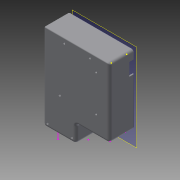
# Autodesk Inventor part: arduino-holder
Saved by Autodesk Inventor 2014 (Build 180170000, 170)
## iProperties
Created: 2017-08-03
Part Number: arduino-holder
Material: 一般
Document SubType Name: Modeling
Designer: hide
Density: 1 g/cm^3
Appearance: 既定
Author: hide
Autodesk Inventor part; units mm, degrees
ref_plane "YZ Plane" through (0, 0, 0) normal (1, 0, 0) x (0, 1, 0)
ref_plane "XY Plane" through (0, 0, 0) normal (0, 0, 1) x (1, 0, 0)
sketch "スケッチ1" plane through (0, 0, 0) normal (0, 1, 0) x (-1, 0, 0)
  line L0 (0, 0) -> (73, 0)
  line L1 (73, 0) -> (73, -76.4)
  line L2 (0, -76) -> (0, 0)
  circle A0 centre (21.8, -5) radius 1.3
  circle A1 centre (50, -5) radius 1.3
  circle A2 centre (55, -57) radius 1.3
  circle A3 centre (15, -15) radius 1.3
  circle A4 centre (15, -55) radius 1.3
  line L3 (4.5, -3) -> (58, -3)
  line L4 (58, -3) -> (58, -73)
  line L5 (58, -73) -> (4.5, -73)
  line L6 (4.5, -73) -> (4.5, -3)
  line L7 (73, -12.2504) -> (60, -12.2504)
  line L8 (60, -12.2504) -> (60, -2.9504)
  line L9 (60, -2.9504) -> (73, -2.9504)
  line L10 (73, -2.9504) -> (73, -12.2504)
  line L11 (37, -76) -> (37, -95.2)
  line L12 (37, -95.2) -> (73, -95.2)
  line L13 (73, -95.2) -> (73, -76.4)
  line L14 (39, -73.2) -> (71, -73.2)
  line L15 (71, -73.2) -> (71, -93.2)
  line L16 (71, -93.2) -> (39, -93.2)
  line L17 (39, -93.2) -> (39, -73.2)
  circle A5 centre (41.6, -75.8) radius 1.3
  circle A6 centre (41.6, -90.6) radius 1.3
  circle A7 centre (68.4, -75.8) radius 1.3
  circle A8 centre (68.4, -90.6) radius 1.3
  line L18 (0, -76) -> (37, -76)
  dimension "d0" = 0
  dimension "d1" = 28.2
  dimension "d2" = 5
  dimension "d3" = 2.6
  dimension "d4" = 2.6
  dimension "d5" = 2.6
  dimension "d13" = 52
  dimension "d14" = 0
  dimension "d15" = 40
  dimension "d16" = 2.6
  dimension "d17" = 2.6
  dimension "d20" = 70
  dimension "d21" = 2
  dimension "d22" = 53.5
  dimension "d23" = 3
  dimension "d24" = 9.3
  dimension "d31" = 15
  dimension "d32" = 15
  dimension "d92" = 4.5
  dimension "d93" = 3
  dimension "d94" = 15
  dimension "d110" = 76.4
  dimension "d111" = 32
  dimension "d114" = 2
  dimension "d115" = 2
  dimension "d118" = 2.6
  dimension "d121" = 2.6
  dimension "d122" = 2.6
  dimension "d123" = 2.6
  dimension "d124" = 2.6
  dimension "d125" = 2.6
  dimension "d126" = 2.6
  dimension "d127" = 2.6
  dimension "d128" = 2.6
  dimension "d129" = 2.6
  dimension "d134" = 13
  dimension "d135" = 2
  dimension "d147" = 3
  dimension "d148" = 0.2
  dimension "d149" = 20
  dimension "d150" = 2.6
  dimension "d151" = 2.6
  constraints: 38 end point, 9 centre point, 8 parallel, 5 perpendicular, 4 horizontal, 1 point on line
  measures "d0" vertical distance of A1.centre A0.centre
  measures "d1" distance of A0.centre A1.centre
  measures "d2" horizontal distance of A2.centre A1.centre
  measures "d3" diameter of A0
  measures "d4" diameter of A1
  measures "d5" diameter of A2
  measures "d13" vertical distance of A2.centre A1.centre
  measures "d14" horizontal distance of A4.centre A3.centre
  measures "d15" distance of A3.centre A4.centre
  measures "d16" diameter of A3
  measures "d17" diameter of A4
  measures "d20" distance of L3.end L4.end
  measures "d21" distance from line of L3 A1.centre
  measures "d22" distance between parallel lines of L4 L6
  measures "d23" distance from line of L4 A2.centre
  measures "d24" distance between parallel lines of L7 L9
  measures "d31" distance from line of L0 A3.centre
  measures "d32" distance from line of L2 A3.centre
  measures "d92" distance between parallel lines of L2 L6
  measures "d93" distance between parallel lines of L0 L3
  measures "d94" distance between parallel lines of L1 L4
  measures "d110" distance of L0.end L1.end
  measures "d111" distance between parallel lines of L15 L17
  measures "d114" distance between parallel lines of L16 L12
  measures "d115" distance between parallel lines of L17 L11
  measures "d118" distance from line of L17 A5.centre
  measures "d121" distance from line of L15 A7.centre
  measures "d122" distance from line of L15 A8.centre
  measures "d123" distance from line of L16 A8.centre
  measures "d124" distance from line of L16 A6.centre
  measures "d125" distance from line of L17 A6.centre
  measures "d126" diameter of A7
  measures "d127" diameter of A5
  measures "d128" diameter of A6
  measures "d129" diameter of A8
  measures "d134" distance between parallel lines of L10 L8
  measures "d135" distance between parallel lines of L13 L15
  measures "d147" distance between parallel lines of L5 L18
  measures "d148" distance between parallel lines of L5 L14
  measures "d149" distance of L14.end L15.end
  measures "d150" distance from line of L14 A5.centre
  measures "d151" distance from line of L14 A7.centre
extrude "押し出し1" add sketch "スケッチ1" along normal blind 2 contours L0 L1 L9 L8 L7 L13 L12 L11 L18 L2 | L1 L7 L8 L9 | L3 L4 L5 L6 | L14 L15 L16 L17 | A5 | A7
sketch "スケッチ2" plane through (0, 2, 0) normal (0, 1, 0) x (1, 0, 0)
  circle A0 centre (-55, 57) radius 1.3 projected
  circle A1 centre (-50, 5) radius 1.3 projected
  circle A2 centre (-21.8, 5) radius 1.3 projected
  circle A3 centre (-55, 57) radius 2.7
  circle A4 centre (-50, 5) radius 2.7
  circle A5 centre (-21.8, 5) radius 2.7
  circle A6 centre (-15, 55) radius 1.3 projected
  circle A7 centre (-15, 15) radius 1.3 projected
  circle A8 centre (-15, 55) radius 2.8
  circle A9 centre (-15, 15) radius 2.8
  circle A10 centre (-41.6, 79) radius 1.3 projected
  circle A11 centre (-41.6, 90.6) radius 1.3 projected
  circle A12 centre (-68.4, 79) radius 1.3 projected
  circle A13 centre (-68.4, 90.6) radius 1.3 projected
  circle A14 centre (-68.4, 90.6) radius 2.7
  circle A15 centre (-68.4, 79) radius 2.7
  circle A16 centre (-41.6, 79) radius 2.7
  circle A17 centre (-41.6, 90.6) radius 2.7
  dimension "d8" = 1.4
  dimension "d9" = 1.4
  dimension "d10" = 1.4
  dimension "d18" = 1.5
  dimension "d19" = 1.5
  dimension "d130" = 1.4
  dimension "d131" = 1.4
  dimension "d132" = 1.4
  dimension "d133" = 1.4
  constraints: 9 centre point, 9 coincident
  measures "d8" radial gap between concentric circles of A3 A0
  measures "d9" radial gap between concentric circles of A1 A4
  measures "d10" radial gap between concentric circles of A5 A2
  measures "d18" radial gap between concentric circles of A8 A6
  measures "d19" radial gap between concentric circles of A7 A9
  measures "d130" radial gap between concentric circles of A14 A13
  measures "d131" radial gap between concentric circles of A12 A15
  measures "d132" radial gap between concentric circles of A16 A10
  measures "d133" radial gap between concentric circles of A17 A11
extrude "押し出し2" add sketch "スケッチ2" along normal blind 7 contours A3 | A4 | A5 | A14 | A17
sketch "スケッチ3" plane through (0, 2, 0) normal (0, 1, 0) x (1, 0, 0)
  line L0 (-73, 0) -> (0, 0) projected
  line L1 (0, 0) -> (0, 76) projected
  line L2 (0, 75.4) -> (0, 0)
  line L3 (0, 0) -> (-60, 0)
  line L4 (-38.3, 75.1) -> (-1.3, 75.1)
  line L5 (-1.3, 75.1) -> (-1.3, 1.3)
  line L6 (-1.3, 1.3) -> (-70.631, 1.3)
  line L7 (-73, 95.2) -> (-70.631, 95.2)
  line L8 (-73, 78.8) -> (-73, 95.2)
  line L9 (-70.631, 95.2) -> (-37, 95.2)
  line L10 (-24, 75.1) -> (-38.3, 75.1)
  line L11 (-73, 95.2) -> (-73, 0) projected
  line L12 (-73, 95.2) -> (-71.7, 95.2)
  line L13 (-71.7, 95.2) -> (-71.7, 0)
  line L14 (-71.7, 0) -> (-73, 0)
  line L15 (-73, 0) -> (-73, 95.2)
  line L16 (-73, 0) -> (0, 0)
  line L17 (0, 0) -> (0, 1.3)
  line L18 (0, 1.3) -> (-73, 1.3)
  line L19 (-73, 1.3) -> (-73, 0)
  line L20 (0, 0) -> (-1.3, 0)
  line L21 (-1.3, 0) -> (-1.3, 76)
  line L22 (-1.3, 76) -> (0, 76)
  line L23 (0, 76) -> (0, 0)
  line L24 (-38.3, 76) -> (-38.3, 74.7)
  line L25 (-38.3, 74.7) -> (0, 74.7)
  line L26 (0, 74.7) -> (0, 76)
  line L27 (-37, 95.2) -> (-38.9, 95.2)
  line L28 (-38.3, 74.7) -> (-36.4, 74.7)
  line L29 (-37, 95.2) -> (-73, 95.2)
  line L30 (-73, 95.2) -> (-73, 93.9)
  line L31 (-73, 93.9) -> (-37, 93.9)
  line L32 (-37, 93.9) -> (-37, 95.2)
  circle A0 centre (-41.6, 90.6) radius 2.7 projected
  circle A1 centre (-21.8, 5) radius 2.7 projected
  circle A2 centre (-55, 57) radius 2.7 projected
  circle A3 centre (-50, 5) radius 2.7 projected
  circle A4 centre (-68.4, 90.6) radius 2.7 projected
  circle A5 centre (-15, 55) radius 1.3 projected
  line L33 (-73, 0) -> (0, 0) projected
  line L34 (0, 0) -> (0, 76) projected
  line L35 (-37, 76) -> (-37, 95.2) projected
  line L36 (-37, 95.2) -> (-73, 95.2) projected
  line L37 (-73, 95.2) -> (-73, 0) projected
  line L38 (-37, 95.2) -> (-38.3, 95.2)
  line L39 (-38.3, 95.2) -> (-38.3, 74.7)
  line L40 (-38.3, 74.7) -> (-37, 74.7)
  line L41 (-37, 74.7) -> (-37, 95.2)
  line L42 (0, 76) -> (-37, 76) projected
  line L43 (-38.3, 74.7) -> (0, 74.7)
  line L44 (0, 74.7) -> (0, 76)
  line L45 (0, 76) -> (-38.3, 76)
  line L46 (-38.3, 76) -> (-38.3, 74.7)
  dimension "d27" = 1.3
  dimension "d28" = 1.3
  dimension "d136" = 1.3
  dimension "d137" = 1.3
  dimension "d138" = 1.3
  dimension "d139" = 1.3
  dimension "d141" = 1.3
  dimension "d152" = 0
  dimension "d153" = 1.3
  constraints: 76 end point, 15 parallel, 10 horizontal, 7 perpendicular, 4 point on line
  measures "d27" distance between parallel lines of L1 L5
  measures "d28" distance between parallel lines of L6 L0
  measures "d136" distance between parallel lines of L29 L31
  measures "d137" distance between parallel lines of L11 L13
  measures "d138" distance between parallel lines of L18 L0
  measures "d139" distance between parallel lines of L2 L21
  measures "d141" distance between parallel lines of L41 L39
  measures "d152" distance between parallel lines of L22 L42
  measures "d153" distance between parallel lines of L45 L43
extrude "押し出し3" add sketch "スケッチ3" along normal blind 25 contours L11 L18 L13 L0 | L13 L18 L6 L21 L0 | L11 L8 L31 L13 L18 | L21 L18 L1 L0 | L31 L8 L7 L13 | L13 L7 L9 L39 L31 | L5 L25 L1 L18 | L39 L9 L32 L31 | L31 L35 L45 L39 | L25 L41 L4 L5 | L5 L21 L22 L1 L25 | L45 L41 L4 L24 | L4 L41 L42 L21 | L4 L41 L25 L24
sketch "スケッチ4" plane through (0, 2, 0) normal (0, 1, 0) x (1, 0, 0)
  line L0 (-1.3, 1.3) -> (-1.3, 75.1) projected
  line L1 (-1.3, 75.1) -> (-38.3, 75.1) projected
  line L2 (-58.7, 102.1) -> (-58.7, 1.3) projected
  line L3 (-58.7, 1.3) -> (-1.3, 1.3) projected
  circle A0 centre (-20, 15) radius 2.8 projected
  circle A1 centre (-21.8, 5) radius 2.7 projected
  circle A2 centre (-55, 57) radius 2.7 projected
  circle A3 centre (-50, 5) radius 2.7 projected
  circle A4 centre (-20, 55) radius 2.8 projected
  point P0 (-58.7, 85.7)
  point P1 (0, 0)
  point P2 (-25.3, 85.7)
  point P3 (-58.7, 87)
  constraints: 1 other
sketch "スケッチ5" plane through (0, 2, 0) normal (0, 1, 0) x (1, 0, 0)
  circle A0 centre (-15, 55) radius 1.3 projected
  circle A1 centre (-15, 15) radius 1.3 projected
  circle A2 centre (-15, 55) radius 3
  circle A3 centre (-15, 15) radius 3
  point P0 (0, 0)
  dimension "d33" = 6
  dimension "d34" = 6
  constraints: 2 centre point, 2 coincident
  measures "d33" diameter of A2
  measures "d34" diameter of A3
extrude "押し出し4" add sketch "スケッチ5" along normal blind 5
sketch "スケッチ7" plane through (0, 2, 0) normal (0, 1, 0) x (1, 0, 0)
  line L0 (-58.7, 1.3) -> (-1.3, 1.3) projected
  line L1 (-58.7, 1.3) -> (-48, 1.3)
  line L2 (-48, 1.3) -> (-48, 11.3)
  line L3 (-48, 11.3) -> (-58.7, 11.3)
  line L4 (-58.7, 11.3) -> (-58.7, 1.3)
  line L5 (-58.7, 1.3) -> (-46.5, 1.3)
  line L6 (-46.5, 1.3) -> (-46.5, 12.8)
  line L7 (-46.5, 12.8) -> (-58.7, 12.8)
  line L8 (-58.7, 12.8) -> (-58.7, 1.3)
  line L9 (-71.7, 1.3) -> (-61, 1.3)
  line L10 (-61, 1.3) -> (-61, 11.3)
  line L11 (-61, 11.3) -> (-71.7, 11.3)
  line L12 (-71.7, 11.3) -> (-71.7, 1.3)
  line L13 (-71.7, 1.3) -> (-59.5, 1.3)
  line L14 (-59.5, 1.3) -> (-59.5, 12.8)
  line L15 (-59.5, 12.8) -> (-71.7, 12.8)
  line L16 (-71.7, 12.8) -> (-71.7, 1.3)
  point P0 (0, 0)
  dimension "d43" = 10.7
  dimension "d44" = 10
  dimension "d45" = 1.5
  dimension "d46" = 1.5
  dimension "d143" = 10
  dimension "d144" = 1.5
  dimension "d145" = 10.7
  dimension "d146" = 1.5
  constraints: 32 end point, 8 parallel, 4 horizontal, 4 perpendicular
  measures "d43" distance between parallel lines of L2 L4
  measures "d44" distance between parallel lines of L0 L3
  measures "d45" distance between parallel lines of L7 L3
  measures "d46" distance between parallel lines of L6 L2
  measures "d143" distance between parallel lines of L11 L13
  measures "d144" distance between parallel lines of L15 L11
  measures "d145" distance between parallel lines of L16 L10
  measures "d146" distance between parallel lines of L10 L14
extrude "押し出し6" add sketch "スケッチ7" along normal blind 11 contours L10 L11 L16 L15 L14 L13
sketch "スケッチ8" plane through (0, 2, 0) normal (0, 1, 0) x (1, 0, 0)
  line L0 (-58.7, 11.3) -> (-65.1062, 11.3)
  line L1 (-65.1062, 11.3) -> (-65.1062, 1.3)
  line L2 (-65.1062, 1.3) -> (-58.7, 1.3)
  line L3 (-58.7, 1.3) -> (-48, 1.3) projected
  line L4 (-71.7, 11.3) -> (-77.9031, 11.3)
  line L5 (-77.9031, 11.3) -> (-77.9031, 1.3)
  line L6 (-77.9031, 1.3) -> (-71.7, 1.3)
  line L7 (-71.7, 1.3) -> (-71.7, 11.3)
  point P0 (0, 0)
  dimension "d54" = 0
  constraints: 14 end point, 3 parallel, 2 horizontal, 2 perpendicular
  measures "d54" distance between parallel lines of L2 L3
extrude "押し出し7" cut sketch "スケッチ8" against normal blind 11 and the other way blind 11.5
fillet "フィレット1" radius 5 2 edges at (-66.35, 2, -11.3) (-66.35, 2, -1.3)
ref_plane "作業平面1" through (0, 26.8, 0) normal (0, 1, 0) x (-1, 0, 0)
sketch "スケッチ9" plane through (0, 26.8, 0) normal (0, 1, 0) x (-1, 0, 0)
  circle A0 centre (3, -3) radius 0.75
  circle A1 centre (3, -3) radius 2.5
  circle A2 centre (70.0026, -50.581) radius 0.75
  circle A3 centre (70.0026, -50.581) radius 2.5
  line L0 (7.986, -75.1) -> (20.986, -75.1) projected
  line L1 (1.3, -1.3) -> (71.7, -1.3) projected
  line L2 (1.3, -75.1) -> (1.3, -1.3) projected
  circle A4 centre (3, -73.4) radius 0.75
  circle A5 centre (3, -73.4) radius 2.5
  circle A6 centre (70.0026, -3) radius 0.75
  circle A7 centre (70.0026, -3) radius 2.5
  line L3 (7.986, -75.1) -> (1.3, -75.1) projected
  line L4 (58.7, -102.1) -> (38.3, -102.1) projected
  line L5 (0, -76) -> (37, -76) projected
  line L6 (37, -76) -> (37, -95.2) projected
  line L7 (37, -95.2) -> (73, -95.2) projected
  line L8 (73, -95.2) -> (73, 0) projected
  line L9 (73, 0) -> (0, 0) projected
  line L10 (0, 0) -> (0, -76) projected
  line L11 (1.3, -74.7) -> (1.3, -1.3) projected
  line L12 (71.7, -1.3) -> (71.7, -93.9) projected
  line L13 (71.7, -93.9) -> (38.3, -93.9) projected
  line L14 (1.3, -1.3) -> (71.7, -1.3) projected
  line L15 (38.3, -93.9) -> (38.3, -74.7) projected
  line L16 (38.3, -74.7) -> (1.3, -74.7) projected
  point P0 (58.7, -85.7)
  point P1 (25.3, -85.7)
  point P2 (58.7, -87)
  dimension "d56" = 1.5
  dimension "d57" = 5
  dimension "d58" = 1.5
  dimension "d59" = 5
  dimension "d62" = 1.7
  dimension "d63" = 1.7
  dimension "d100" = 5
  dimension "d101" = 1.5
  dimension "d102" = 1.5
  dimension "d103" = 5
  dimension "d104" = 1.7
  dimension "d105" = 1.7
  dimension "d106" = 1.7
  constraints: 8 centre point, 4 coincident, 1 other
  measures "d56" diameter of A0
  measures "d57" diameter of A1
  measures "d58" diameter of A2
  measures "d59" diameter of A3
  measures "d62" distance from line of L1 A0.centre
  measures "d63" distance from line of L2 A0.centre
  measures "d100" diameter of A7
  measures "d101" diameter of A6
  measures "d102" diameter of A4
  measures "d103" diameter of A5
  measures "d104" distance from line of L2 A4.centre
  measures "d105" distance from line of A4.centre L3
  measures "d106" distance from line of L1 A6.centre
extrude "押し出し8" add sketch "スケッチ9" against normal blind 8 contours A1 L2 L1 | L1 L2 A1 | A7 L12 L1 | L1 L12 A7 | A5 L16 L2 | L2 L3 A5 | L16 A5 L3 L2 | L12 A3 | A3 L12
sketch "スケッチ11" plane through (0, 18.8, 0) normal (0, -1, 0) x (1, 0, 0)
  line L0 (-58.7, -3) -> (-58.7, -1.3) projected
  line L1 (-1.3, -75.1) -> (-5.5, -75.1) projected
  circle A0 centre (-70.0026, -50.581) radius 2.5 projected
  circle A1 centre (-70.0026, -50.581) radius 0.75 projected
  point P0 (-72.5026, -50.581)
  point P1 (-58.7, -85.7)
  point P2 (-72.5026, -50.581)
  point P3 (0, 0)
  point P4 (-5.5, -73.4)
  point P5 (-72.5026, -50.581)
  point P6 (-72.5026, -3)
  point P7 (-72.5026, -50.581)
  point P8 (-58.7, -1.3)
  constraints: 2 other
fillet "フィレット4" radius 3 12 edges at (0, 13.5, 0) (0, 0, -38) (-73, 0, -0.65) (-73, 0, -53.25) (-73, 13.5, 0) (-55, 0, -95.2) (-37, 0, -85.6) (-37, 13.5, -95.2) (-73, 13.5, -95.2) (-18.5, 0, -76) (0, 13.5, -76) (-37, 13.5, -76)
fillet "フィレット5" radius 1 3 edges at (-71.3964, 0.3448, -0.3448) (-0.8787, 0.8787, -0.8787) (-36.5, 0, 0)
sketch "スケッチ15" plane through (0, 3, -73.4) normal (1, 0, 0) x (0, 0, -1)
  line L0 (-73.4, 24) -> (-0.4, 24) projected
  line L1 (-73.4, 24) -> (-73.4, -2) projected
  line L2 (-64.5, 24) -> (-50.5, 24)
  line L3 (-50.5, 24) -> (-50.5, 18.8)
  line L4 (-50.5, 18.8) -> (-64.5, 18.8)
  line L5 (-64.5, 18.8) -> (-64.5, 24)
  point P0 (0, 24)
  point P1 (-73.4, -3)
  point P2 (2.6, 24)
  dimension "d95" = 14
  dimension "d96" = 5.2
  dimension "d97" = 8.9
  constraints: 8 end point, 2 parallel, 1 horizontal, 1 perpendicular, 1 point on line
  measures "d95" distance of L3.end L4.end
  measures "d96" distance of L4.end L2.start
  measures "d97" distance between parallel lines of L1 L5
extrude "押し出し12" cut sketch "スケッチ15" against normal blind 10
fillet "フィレット8" radius 1 6 edges at (-38.3, 14.5, -93.9) (-1.3, 10.4, -74.7) (-71.7, 14.5, -93.9) (-71.7, 16.15, -1.3) (-1.3, 10.4, -1.3) (-38.3, 14.5, -74.7)
sketch "スケッチ16" plane through (-3, 3, -76) normal (0, 0, -1) x (-1, 0, 0)
  line L0 (0, 24) -> (31, 24) projected
  line L1 (-3, 24) -> (-3, 0) projected
  line L2 (9, 24) -> (22, 24)
  line L3 (22, 24) -> (22, 7)
  line L4 (22, 7) -> (9, 7)
  line L5 (9, 7) -> (9, 24)
  point P0 (-3, -3)
  dimension "d155" = 12
  dimension "d156" = 13
  dimension "d157" = 17
  constraints: 8 end point, 2 parallel, 1 horizontal, 1 perpendicular, 1 point on line
  measures "d155" distance between parallel lines of L5 L1
  measures "d156" distance between parallel lines of L3 L5
  measures "d157" distance of L4.end L2.start
extrude "押し出し13" cut sketch "スケッチ16" against normal blind 3
sketch "スケッチ18" plane through (-68.4, 9, -90.6) normal (0, 1, 0) x (1, 0, 0)
  circle A0 centre (0, 0) radius 1.3 projected
  circle A1 centre (0, 0) radius 2.7 projected
  circle A2 centre (26.8, 0) radius 1.3 projected
  circle A3 centre (26.8, 0) radius 2.7 projected
  point P0 (68.4, -90.6)
extrude "押し出し14" add sketch "スケッチ18" along normal blind 6.5
draft "面の勾配5" angle 5 pull direction (0, 1, 0) faces at (-65.7088, 11, -90.3827) fixed edges at (-71.1, 15.5, -90.6)
draft "面の勾配6" angle 5 pull direction (0, 1, 0) faces at (-38.935, 6.5, -90.1669) fixed edges at (-44.3, 15.5, -90.6)
equation "\"d4\" = d3"
equation "\"d5\" = d3"
equation "\"d17\" = d16"
equation "\"d9\" = d8"
equation "\"d10\" = d8"
equation "\"d19\" = d18"
equation "\"d27\" = d25"
equation "\"d28\" = d25"
equation "\"d46\" = d45"
equation "\"d63\" = d62"
equation "\"d100\" = d57"
equation "\"d101\" = d56"
equation "\"d102\" = d56"
equation "\"d103\" = d57"
equation "\"d104\" = d61"
equation "\"d105\" = d60"
equation "\"d106\" = d62"
equation "\"d60\" = d62"
equation "\"d61\" = d60"
equation "\"d25\" = 1.3"
